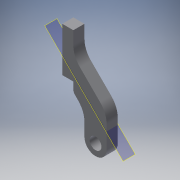
# Autodesk Inventor part: Mirror
Saved by Autodesk Inventor 2016 (Build 200138000, 138)
## iProperties
Created: 2013-12-15
Part Number: Mirror
Material: Generic
Document SubType Name: Modeling
Designer: John
Density: 1 g/cm^3
Appearance: Default
Author: John
Autodesk Inventor part; units mm, degrees
ref_plane "YZ Plane" through (0, 0, 0) normal (1, 0, 0) x (0, 1, 0)
ref_plane "XZ Plane" through (0, 0, 0) normal (0, 1, 0) x (-1, 0, 0)
ref_plane "XY Plane" through (0, 0, 0) normal (0, 0, 1) x (1, 0, 0)
sketch "Sketch1" plane through (0, 0, 0) normal (0, 0, 1) x (1, 0, 0)
  line L0 (0, 0) -> (6.35, 0)
  line L1 (6.35, 0) -> (6.35, 25.4)
  line L2 (6.35, 25.4) -> (0, 25.4)
  line L3 (0, 25.4) -> (0, 0)
  line L4 (6.35, 0) -> (6.35, -5.2605)
  line L5 (6.35, -5.2605) -> (12.7, -11.6105)
  line L6 (12.7, -11.6105) -> (12.7, -24.3105)
  arc A0 (12.7, -24.3105) -> (25.4, -24.3105) centre (19.05, -24.3105) ccw
  line L7 (25.4, -24.3105) -> (25.4, -6.35)
  line L8 (25.4, -6.35) -> (6.35, 12.7)
  dimension "d0" = 6.35
  dimension "d1" = 25.4
  dimension "d2" = 6.35
  dimension "d3" = 12.7
  dimension "d4" = 12.7
  dimension "d5" = 45
  constraints: 18 end point, 6 parallel, 2 midpoint, 2 point on circle, 2 tangent, 1 centre point, 1 horizontal, 1 perpendicular, 1 point on line
  measures "d0" distance of L2.end L1.end
  measures "d1" distance of L1.end L0.end
  measures "d2" radius of A0
  measures "d3" distance between parallel lines of L8 L5
  measures "d4" distance from line of A0.centre L1
  measures "d5" angle of L8 L1
extrude "Extrusion1" add sketch "Sketch1" along normal blind 6.35
fillet "Fillet1" radius 3.175 1 edges at (6.35, -5.2605, 3.175)
fillet "Fillet2" radius 12.7 3 edges at (12.7, -11.6105, 3.175) (25.4, -6.35, 3.175) (6.35, 12.7, 3.175)
sketch "Sketch2" plane through (0, 0, 6.35) normal (0, 0, 1) x (1, 0, 0)
  arc A0 (12.7, -24.3105) -> (25.4, -24.3105) centre (19.05, -24.3105) ccw projected
hole "Hole1" at (19.05, -24.3105, 6.35) direction (0, 0, -1) diameter 6.7564 end through all clearance for "Socket Head Cap Screw" size "1/4" standard "Ansi Unified Screw Threads"
ref_plane "Work Plane1" through (11.7701, -1.7003, 6.35) normal (-0.7071, -0.7071, 0) x (-0.7071, 0.7071, 0)
body "Solid1"
